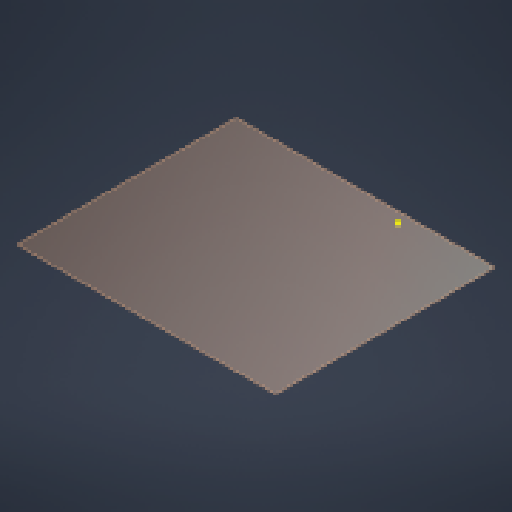
# Autodesk Inventor part: Cover Right
Saved by Autodesk Inventor 2026.1 (Build 301233020, 233B)
## iProperties
Created: 2026-06-25
Part Number: Cover Right
Material: Generic
Document SubType Name: Modeling
Designer: Bahaa
Mass: 5.68876 g
Surface Area: 120.492 cm^2
Volume: 5.68876 cm^3
Density: 1 g/cm^3
Appearance: Black PLA
Author: Bahaa
Autodesk Inventor part; units mm, degrees
ref_plane "YZ Plane" through (0, 0, 0) normal (1, 0, 0) x (0, 1, 0)
ref_plane "XZ Plane" through (0, 0, 0) normal (0, 1, 0) x (-1, 0, 0)
ref_plane "XY Plane" through (0, 0, 0) normal (0, 0, 1) x (1, 0, 0)
ref_plane "Work Plane1" through (0, 0, 0) normal (0, 0, 1) x (1, 0, 0)
sketch "Sketch1" plane through (0, 0, 0) normal (0, 0, 1) x (1, 0, 0)
  circle A0 centre (-1.9788, -172.3545) radius 2.85 projected
  circle A1 centre (36.7695, -114.5513) radius 1.6 projected
  circle A2 centre (-114.5513, -114.5513) radius 1.6 projected
  circle A3 centre (-114.5513, -36.7695) radius 1.6 projected
  circle A4 centre (36.7696, -36.7696) radius 1.6 projected
  circle A5 centre (-120.2082, -108.8944) radius 2.85 projected
  circle A6 centre (-120.2082, -42.4264) radius 2.85 projected
  circle A7 centre (42.4264, -42.4264) radius 2.85 projected
  circle A8 centre (42.4264, -108.8944) radius 2.85 projected
  circle A9 centre (0, -151.3209) radius 2.85 projected
  circle A10 centre (-77.7818, -151.3208) radius 2.85 projected
  arc A11 (3.1213, -2.5355) -> (3.3245, -2.9609) centre (3.2981, -2.7123) ccw projected
  arc A12 (4.9497, -3.5355) -> (3.3245, -2.9609) centre (3.5355, -4.9497) ccw projected
  line L0 (4.9497, -3.5355) -> (33.234, -31.8198) projected
  arc A13 (33.234, -34.6482) -> (33.234, -31.8198) centre (31.8198, -33.234) ccw projected
  line L1 (33.234, -34.6482) -> (32.5269, -35.3553) projected
  arc A14 (32.5269, -35.3553) -> (32.5269, -38.1838) centre (33.9411, -36.7696) ccw projected
  line L2 (32.5269, -38.1838) -> (41.0122, -46.669) projected
  arc A15 (41.0122, -46.669) -> (43.8406, -46.669) centre (42.4264, -45.2548) ccw projected
  line L3 (43.8406, -46.669) -> (50.8531, -39.6566) projected
  arc A16 (54.1372, -40.3613) -> (50.8531, -39.6566) centre (52.2673, -41.0708) ccw projected
  arc A17 (54.1372, -110.9596) -> (54.1372, -40.3613) centre (-38.8909, -75.6604) ccw projected
  arc A18 (50.8531, -111.6643) -> (54.1372, -110.9596) centre (52.2673, -110.25) ccw projected
  line L4 (50.8531, -111.6643) -> (43.8406, -104.6518) projected
  arc A19 (43.8406, -104.6518) -> (41.0122, -104.6518) centre (42.4264, -106.066) ccw projected
  line L5 (41.0122, -104.6518) -> (32.5269, -113.1371) projected
  arc A20 (32.5269, -113.1371) -> (32.5269, -115.9655) centre (33.9411, -114.5513) ccw projected
  line L6 (32.5269, -115.9655) -> (33.234, -116.6726) projected
  arc A21 (33.234, -119.501) -> (33.234, -116.6726) centre (31.8198, -118.0868) ccw projected
  line L7 (33.234, -119.501) -> (4.9497, -147.7853) projected
  arc A22 (2.1213, -147.7853) -> (4.9497, -147.7853) centre (3.5355, -146.3711) ccw projected
  line L8 (2.1213, -147.7853) -> (1.4142, -147.0782) projected
  arc A23 (1.4142, -147.0782) -> (-1.4142, -147.0782) centre (0, -148.4924) ccw projected
  line L9 (-1.4142, -147.0782) -> (-9.8995, -155.5635) projected
  arc A24 (-9.8995, -155.5635) -> (-9.8995, -158.3919) centre (-8.4853, -156.9777) ccw projected
  line L10 (-9.8995, -158.3919) -> (-2.8871, -165.4044) projected
  arc A25 (-3.5917, -168.6885) -> (-2.8871, -165.4044) centre (-4.3013, -166.8186) ccw projected
  arc A26 (-21.3624, -173.6043) -> (-3.5917, -168.6885) centre (-38.8909, -75.6604) ccw projected
  arc A27 (-24.8909, -170.6512) -> (-21.3624, -173.6043) centre (-21.8909, -170.6512) ccw projected
  line L11 (-24.8909, -107.6604) -> (-24.8909, -170.6512) projected
  arc A28 (-24.8909, -107.6604) -> (-27.8909, -104.6604) centre (-27.8909, -107.6604) ccw projected
  line L12 (-49.8909, -104.6604) -> (-27.8909, -104.6604) projected
  arc A29 (-49.8909, -104.6604) -> (-52.8909, -107.6604) centre (-49.8909, -107.6604) ccw projected
  line L13 (-52.8909, -170.6512) -> (-52.8909, -107.6604) projected
  arc A30 (-56.4194, -173.6043) -> (-52.8909, -170.6512) centre (-55.8909, -170.6512) ccw projected
  arc A31 (-74.19, -168.6885) -> (-56.4194, -173.6043) centre (-38.8909, -75.6604) ccw projected
  arc A32 (-74.8947, -165.4044) -> (-74.19, -168.6885) centre (-73.4805, -166.8186) ccw projected
  line L14 (-74.8947, -165.4044) -> (-67.8823, -158.3919) projected
  arc A33 (-67.8823, -158.3919) -> (-67.8823, -155.5635) centre (-69.2965, -156.9777) ccw projected
  line L15 (-67.8823, -155.5635) -> (-76.3675, -147.0782) projected
  arc A34 (-76.3675, -147.0782) -> (-79.196, -147.0782) centre (-77.7817, -148.4924) ccw projected
  line L16 (-79.196, -147.0782) -> (-79.9031, -147.7853) projected
  arc A35 (-82.7315, -147.7853) -> (-79.9031, -147.7853) centre (-81.3173, -146.3711) ccw projected
  line L17 (-82.7315, -147.7853) -> (-111.0158, -119.501) projected
  arc A36 (-111.0158, -116.6726) -> (-111.0158, -119.501) centre (-109.6016, -118.0868) ccw projected
  line L18 (-111.0158, -116.6726) -> (-110.3087, -115.9655) projected
  arc A37 (-110.3087, -115.9655) -> (-110.3087, -113.1371) centre (-111.7229, -114.5513) ccw projected
  line L19 (-110.3087, -113.1371) -> (-118.794, -104.6518) projected
  arc A38 (-118.794, -104.6518) -> (-121.6224, -104.6518) centre (-120.2082, -106.066) ccw projected
  line L20 (-121.6224, -104.6518) -> (-128.6348, -111.6642) projected
  arc A39 (-131.9189, -110.9596) -> (-128.6348, -111.6642) centre (-130.049, -110.25) ccw projected
  arc A40 (-138.0344, -84.0758) -> (-131.9189, -110.9596) centre (-38.8909, -75.6604) ccw projected
  arc A41 (-138.0344, -84.0758) -> (-139.0308, -83.1604) centre (-139.0308, -84.1604) ccw projected
  line L21 (-139.0308, -83.1604) -> (-143.8909, -83.1604) projected
  arc A42 (-144.8909, -82.1604) -> (-143.8909, -83.1604) centre (-143.8909, -82.1604) ccw projected
  line L22 (-144.8909, -82.1604) -> (-144.8909, -69.1604) projected
  arc A43 (-143.8909, -68.1604) -> (-144.8909, -69.1604) centre (-143.8909, -69.1604) ccw projected
  line L23 (-143.8909, -68.1604) -> (-139.0308, -68.1604) projected
  arc A44 (-139.0308, -68.1604) -> (-138.0344, -67.245) centre (-139.0308, -67.1604) ccw projected
  arc A45 (-131.9189, -40.3613) -> (-138.0344, -67.245) centre (-38.8909, -75.6604) ccw projected
  arc A46 (-128.6348, -39.6566) -> (-131.9189, -40.3613) centre (-130.049, -41.0708) ccw projected
  line L24 (-128.6348, -39.6566) -> (-121.6224, -46.669) projected
  arc A47 (-121.6224, -46.669) -> (-118.7939, -46.669) centre (-120.2082, -45.2548) ccw projected
  line L25 (-118.7939, -46.669) -> (-110.3087, -38.1838) projected
  arc A48 (-110.3087, -38.1838) -> (-110.3087, -35.3553) centre (-111.7229, -36.7696) ccw projected
  line L26 (-110.3087, -35.3553) -> (-111.0158, -34.6482) projected
  arc A49 (-111.0158, -31.8198) -> (-111.0158, -34.6482) centre (-109.6016, -33.234) ccw projected
  line L27 (-111.0158, -31.8198) -> (-82.7315, -3.5355) projected
  arc A50 (-81.1062, -2.9609) -> (-82.7315, -3.5355) centre (-81.3173, -4.9497) ccw projected
  arc A51 (-81.1062, -2.9609) -> (-80.9031, -2.5355) centre (-81.0798, -2.7123) ccw projected
  line L28 (-80.9031, -2.5355) -> (-83.4386, 0) projected
  line L29 (-83.4386, 0) -> (-119.8546, -36.416) projected
  arc A52 (-120.5617, -36.416) -> (-119.8546, -36.416) centre (-120.2082, -36.0624) ccw projected
  line L30 (-120.5617, -36.416) -> (-131.6714, -25.3063) projected
  arc A53 (-131.6714, -25.3063) -> (-134.06, -25.6695) centre (-132.732, -26.367) ccw projected
  arc A54 (-134.06, -25.6695) -> (-134.06, -125.6514) centre (-38.8909, -75.6604) ccw projected
  arc A55 (-134.06, -125.6514) -> (-131.6714, -126.0145) centre (-132.732, -124.9538) ccw projected
  line L31 (-131.6714, -126.0145) -> (-120.5617, -114.9048) projected
  arc A56 (-119.8546, -114.9048) -> (-120.5617, -114.9048) centre (-120.2082, -115.2584) ccw projected
  line L32 (-119.8546, -114.9048) -> (-78.1353, -156.6241) projected
  arc A57 (-78.1353, -157.3312) -> (-78.1353, -156.6241) centre (-78.4889, -156.9777) ccw projected
  line L33 (-78.1353, -157.3312) -> (-89.245, -168.4409) projected
  arc A58 (-89.245, -168.4409) -> (-88.8818, -170.8295) centre (-88.1843, -169.5016) ccw projected
  arc A59 (-88.8818, -170.8295) -> (-52.1373, -182.3412) centre (-38.8909, -75.6604) ccw projected
  arc A60 (-52.1373, -182.3412) -> (-49.8909, -180.3564) centre (-51.8909, -180.3564) ccw projected
  line L34 (-49.8909, -108.6604) -> (-49.8909, -180.3564) projected
  arc A61 (-48.8909, -107.6604) -> (-49.8909, -108.6604) centre (-48.8909, -108.6604) ccw projected
  line L35 (-28.8909, -107.6604) -> (-48.8909, -107.6604) projected
  arc A62 (-27.8909, -108.6604) -> (-28.8909, -107.6604) centre (-28.8909, -108.6604) ccw projected
  line L36 (-27.8909, -108.6604) -> (-27.8909, -180.3564) projected
  arc A63 (-27.8909, -180.3564) -> (-25.6444, -182.3412) centre (-25.8909, -180.3564) ccw projected
  arc A64 (-25.6444, -182.3412) -> (11.1001, -170.8295) centre (-38.8909, -75.6604) ccw projected
  arc A65 (11.1001, -170.8295) -> (11.4632, -168.4409) centre (10.4025, -169.5016) ccw projected
  line L37 (11.4632, -168.4409) -> (0.3535, -157.3313) projected
  arc A66 (0.3535, -156.6242) -> (0.3535, -157.3313) centre (0.7071, -156.9777) ccw projected
  line L38 (0.3535, -156.6242) -> (42.0728, -114.9049) projected
  arc A67 (42.7799, -114.9049) -> (42.0728, -114.9049) centre (42.4264, -115.2584) ccw projected
  line L39 (42.7799, -114.9049) -> (53.8896, -126.0145) projected
  arc A68 (53.8896, -126.0145) -> (56.2782, -125.6514) centre (54.9503, -124.9538) ccw projected
  arc A69 (56.2782, -125.6514) -> (56.2782, -25.6695) centre (-38.8909, -75.6604) ccw projected
  arc A70 (56.2782, -25.6695) -> (53.8896, -25.3064) centre (54.9503, -26.367) ccw projected
  line L40 (53.8896, -25.3064) -> (42.78, -36.416) projected
  arc A71 (42.0729, -36.416) -> (42.78, -36.416) centre (42.4264, -36.0624) ccw projected
  line L41 (42.0729, -36.416) -> (5.6568, 0) projected
  line L42 (5.6568, 0) -> (3.1213, -2.5355) projected
  arc A72 (-22.8909, -107.6604) -> (-27.8909, -102.6604) centre (-27.8909, -107.6604) ccw
  line L43 (-22.8909, -107.6604) -> (-22.8909, -170.6512)
  arc A73 (-22.8909, -170.6512) -> (-21.7147, -171.6356) centre (-21.8909, -170.6512) ccw
  arc A74 (-21.7147, -171.6356) -> (-4.3013, -166.8186) centre (-38.8909, -75.6604) ccw
  line L44 (-4.3013, -166.8186) -> (-11.3137, -159.8061)
  arc A75 (-11.3137, -154.1493) -> (-11.3137, -159.8061) centre (-8.4853, -156.9777) ccw
  line L45 (-11.3137, -154.1493) -> (-2.8284, -145.664)
  arc A76 (2.8284, -145.664) -> (-2.8284, -145.664) centre (0, -148.4924) ccw
  line L46 (2.8284, -145.664) -> (3.5355, -146.3711)
  line L47 (3.5355, -146.3711) -> (31.8198, -118.0868)
  line L48 (31.8198, -118.0868) -> (31.1127, -117.3797)
  arc A77 (31.1127, -111.7229) -> (31.1127, -117.3797) centre (33.9411, -114.5513) ccw
  line L49 (31.1127, -111.7229) -> (39.598, -103.2376)
  arc A78 (45.2548, -103.2376) -> (39.598, -103.2376) centre (42.4264, -106.066) ccw
  line L50 (45.2548, -103.2376) -> (52.2673, -110.25)
  arc A79 (52.2673, -110.25) -> (52.2673, -41.0708) centre (-38.8909, -75.6604) ccw
  line L51 (52.2673, -41.0708) -> (45.2548, -48.0833)
  arc A80 (39.598, -48.0833) -> (45.2548, -48.0833) centre (42.4264, -45.2548) ccw
  line L52 (39.598, -48.0833) -> (31.1127, -39.598)
  arc A81 (31.1127, -33.9411) -> (31.1127, -39.598) centre (33.9411, -36.7696) ccw
  line L53 (31.1127, -33.9411) -> (31.8198, -33.234)
  line L54 (31.8198, -33.234) -> (3.5355, -4.9497)
  arc A82 (1.7071, -1.1213) -> (3.5355, -4.9497) centre (3.2981, -2.7123) ccw
  line L55 (1.7071, -1.1213) -> (5.6568, 2.8284)
  line L56 (5.6568, 2.8284) -> (42.4264, -33.9411)
  line L57 (42.4264, -33.9411) -> (52.4754, -23.8921)
  arc A83 (58.0488, -24.7394) -> (52.4754, -23.8921) centre (54.9503, -26.367) ccw
  arc A84 (58.0488, -126.5815) -> (58.0488, -24.7394) centre (-38.8909, -75.6604) ccw
  arc A85 (52.4754, -127.4287) -> (58.0488, -126.5815) centre (54.9503, -124.9538) ccw
  line L58 (52.4754, -127.4287) -> (42.4264, -117.3797)
  line L59 (42.4264, -117.3797) -> (2.8284, -156.9777)
  line L60 (2.8284, -156.9777) -> (12.8774, -167.0267)
  arc A86 (12.0301, -172.6001) -> (12.8774, -167.0267) centre (10.4025, -169.5016) ccw
  arc A87 (-25.398, -184.3259) -> (12.0301, -172.6001) centre (-38.8909, -75.6604) ccw
  arc A88 (-29.8909, -180.3564) -> (-25.398, -184.3259) centre (-25.8909, -180.3564) ccw
  line L61 (-29.8909, -180.3564) -> (-29.8909, -109.6604)
  line L62 (-29.8909, -109.6604) -> (-47.8909, -109.6604)
  line L63 (-47.8909, -109.6604) -> (-47.8909, -180.3564)
  arc A89 (-52.3838, -184.3259) -> (-47.8909, -180.3564) centre (-51.8909, -180.3564) ccw
  arc A90 (-89.8119, -172.6001) -> (-52.3838, -184.3259) centre (-38.8909, -75.6604) ccw
  arc A91 (-90.6592, -167.0267) -> (-89.8119, -172.6001) centre (-88.1843, -169.5016) ccw
  line L64 (-90.6592, -167.0267) -> (-80.6102, -156.9777)
  line L65 (-80.6102, -156.9777) -> (-120.2082, -117.3797)
  line L66 (-120.2082, -117.3797) -> (-130.2571, -127.4287)
  arc A92 (-135.8306, -126.5814) -> (-130.2571, -127.4287) centre (-132.732, -124.9538) ccw
  arc A93 (-135.8305, -24.7394) -> (-135.8306, -126.5814) centre (-38.8909, -75.6604) ccw
  arc A94 (-130.2571, -23.8921) -> (-135.8305, -24.7394) centre (-132.732, -26.367) ccw
  line L67 (-130.2571, -23.8921) -> (-120.2082, -33.9411)
  line L68 (-120.2082, -33.9411) -> (-83.4386, 2.8284)
  line L69 (-83.4386, 2.8284) -> (-79.4889, -1.1213)
  arc A95 (-81.3173, -4.9497) -> (-79.4889, -1.1213) centre (-81.0798, -2.7123) ccw
  line L70 (-81.3173, -4.9497) -> (-109.6016, -33.234)
  line L71 (-109.6016, -33.234) -> (-108.8945, -33.9411)
  arc A96 (-108.8945, -39.598) -> (-108.8945, -33.9411) centre (-111.7229, -36.7696) ccw
  line L72 (-108.8945, -39.598) -> (-117.3797, -48.0832)
  arc A97 (-123.0366, -48.0832) -> (-117.3797, -48.0832) centre (-120.2082, -45.2548) ccw
  line L73 (-123.0366, -48.0832) -> (-130.049, -41.0708)
  arc A98 (-130.049, -41.0708) -> (-136.0415, -67.4141) centre (-38.8909, -75.6604) ccw
  arc A99 (-139.0308, -70.1604) -> (-136.0415, -67.4141) centre (-139.0308, -67.1604) ccw
  line L74 (-139.0308, -70.1604) -> (-142.8909, -70.1604)
  line L75 (-142.8909, -70.1604) -> (-142.8909, -81.1604)
  line L76 (-142.8909, -81.1604) -> (-139.0308, -81.1604)
  arc A100 (-136.0415, -83.9067) -> (-139.0308, -81.1604) centre (-139.0308, -84.1604) ccw
  arc A101 (-136.0415, -83.9067) -> (-130.049, -110.25) centre (-38.8909, -75.6604) ccw
  line L77 (-130.049, -110.25) -> (-123.0366, -103.2376)
  arc A102 (-117.3797, -103.2376) -> (-123.0366, -103.2376) centre (-120.2082, -106.066) ccw
  line L78 (-117.3797, -103.2376) -> (-108.8945, -111.7229)
  arc A103 (-108.8945, -117.3797) -> (-108.8945, -111.7229) centre (-111.7229, -114.5513) ccw
  line L79 (-108.8945, -117.3797) -> (-109.6016, -118.0868)
  line L80 (-109.6016, -118.0868) -> (-81.3173, -146.3711)
  line L81 (-81.3173, -146.3711) -> (-80.6102, -145.664)
  arc A104 (-74.9533, -145.664) -> (-80.6102, -145.664) centre (-77.7817, -148.4924) ccw
  line L82 (-74.9533, -145.664) -> (-66.4681, -154.1493)
  arc A105 (-66.4681, -159.8061) -> (-66.4681, -154.1493) centre (-69.2965, -156.9777) ccw
  line L83 (-66.4681, -159.8061) -> (-73.4805, -166.8186)
  arc A106 (-73.4805, -166.8186) -> (-56.067, -171.6356) centre (-38.8909, -75.6604) ccw
  arc A107 (-56.067, -171.6356) -> (-54.8909, -170.6512) centre (-55.8909, -170.6512) ccw
  line L84 (-54.8909, -170.6512) -> (-54.8909, -107.6604)
  arc A108 (-49.8909, -102.6604) -> (-54.8909, -107.6604) centre (-49.8909, -107.6604) ccw
  line L85 (-49.8909, -102.6604) -> (-27.8909, -102.6604)
  line L86 (26.5165, -25.1023) -> (18.0312, -33.5876)
  line L87 (30.052, -24.3952) -> (19.4454, -35.0018)
  line L88 (19.4454, -35.0018) -> (-48.2132, -102.6604)
  line L89 (-22.8909, -107.6604) -> (-22.8909, -93.6016)
  line L90 (-22.8909, -93.6016) -> (-22.8909, -183.9852)
  circle A109 centre (-38.8909, -63.6604) radius 1.35 projected
  circle A110 centre (-38.8909, -87.6604) radius 1.35 projected
  arc A111 (-134.1409, -64.6604) -> (-136.1409, -66.6604) centre (-134.1409, -66.6604) ccw projected
  line L91 (-136.1409, -84.6604) -> (-136.1409, -66.6604) projected
  arc A112 (-136.1409, -84.6604) -> (-134.1409, -86.6604) centre (-134.1409, -84.6604) ccw projected
  line L92 (-113.1409, -86.6604) -> (-134.1409, -86.6604) projected
  arc A113 (-111.1409, -88.6604) -> (-113.1409, -86.6604) centre (-113.1409, -88.6604) ccw projected
  line L93 (-111.1409, -89.9104) -> (-111.1409, -88.6604) projected
  arc A114 (-111.1409, -89.9104) -> (-109.1409, -91.9104) centre (-109.1409, -89.9104) ccw projected
  line L94 (-3.8909, -91.9104) -> (-109.1409, -91.9104) projected
  arc A115 (-1.8948, -93.7854) -> (-3.8909, -91.9104) centre (-3.8909, -93.9104) ccw projected
  arc A116 (-1.8948, -93.7854) -> (0.1013, -95.6604) centre (0.1013, -93.6604) ccw projected
  line L95 (45.1169, -95.6604) -> (0.1013, -95.6604) projected
  arc A117 (45.1169, -95.6604) -> (47.113, -93.7854) centre (45.1169, -93.6604) ccw projected
  arc A118 (49.1091, -91.9104) -> (47.113, -93.7854) centre (49.1091, -93.9104) ccw projected
  line L96 (55.1091, -91.9104) -> (49.1091, -91.9104) projected
  arc A119 (55.1091, -91.9104) -> (57.1091, -89.9104) centre (55.1091, -89.9104) ccw projected
  line L97 (57.1091, -57.6604) -> (57.1091, -89.9104) projected
  arc A120 (57.1091, -57.6604) -> (55.1091, -55.6604) centre (55.1091, -57.6604) ccw projected
  line L98 (0.1091, -55.6604) -> (55.1091, -55.6604) projected
  arc A121 (0.1091, -55.6604) -> (-1.887, -57.5354) centre (0.1091, -57.6604) ccw projected
  arc A122 (-3.8831, -59.4104) -> (-1.887, -57.5354) centre (-3.8831, -57.4104) ccw projected
  line L99 (-106.6409, -59.4104) -> (-3.8831, -59.4104) projected
  arc A123 (-106.6409, -59.4104) -> (-108.6409, -61.4104) centre (-106.6409, -61.4104) ccw projected
  line L100 (-108.6409, -62.6604) -> (-108.6409, -61.4104) projected
  arc A124 (-110.6409, -64.6604) -> (-108.6409, -62.6604) centre (-110.6409, -62.6604) ccw projected
  line L101 (-134.1409, -64.6604) -> (-110.6409, -64.6604) projected
  arc A125 (59.1091, -57.6604) -> (55.1091, -53.6604) centre (55.1091, -57.6604) ccw
  line L102 (59.1091, -57.6604) -> (59.1091, -89.9104)
  arc A126 (55.1091, -93.9104) -> (59.1091, -89.9104) centre (55.1091, -89.9104) ccw
  line L103 (55.1091, -93.9104) -> (49.1091, -93.9104)
  arc A127 (45.1169, -97.6604) -> (49.1091, -93.9104) centre (45.1169, -93.6604) ccw
  line L104 (45.1169, -97.6604) -> (0.1013, -97.6604)
  arc A128 (-3.8909, -93.9104) -> (0.1013, -97.6604) centre (0.1013, -93.6604) ccw
  line L105 (-3.8909, -93.9104) -> (-109.1409, -93.9104)
  arc A129 (-113.1409, -89.9104) -> (-109.1409, -93.9104) centre (-109.1409, -89.9104) ccw
  line L106 (-113.1409, -89.9104) -> (-113.1409, -88.6604)
  line L107 (-113.1409, -88.6604) -> (-134.1409, -88.6604)
  arc A130 (-138.1409, -84.6604) -> (-134.1409, -88.6604) centre (-134.1409, -84.6604) ccw
  line L108 (-138.1409, -84.6604) -> (-138.1409, -66.6604)
  arc A131 (-134.1409, -62.6604) -> (-138.1409, -66.6604) centre (-134.1409, -66.6604) ccw
  line L109 (-134.1409, -62.6604) -> (-110.6409, -62.6604)
  line L110 (-110.6409, -62.6604) -> (-110.6409, -61.4104)
  arc A132 (-106.6409, -57.4104) -> (-110.6409, -61.4104) centre (-106.6409, -61.4104) ccw
  line L111 (-106.6409, -57.4104) -> (-3.8831, -57.4104)
  arc A133 (0.1091, -53.6604) -> (-3.8831, -57.4104) centre (0.1091, -57.6604) ccw
  line L112 (0.1091, -53.6604) -> (55.1091, -53.6604)
  point P0 (0, 0)
  point P1 (-22.8909, -93.9104)
  point P2 (-22.8909, -181.9631)
  point P3 (0.7868, -53.6604)
  dimension "d0" = 2
  dimension "d1" = 2
  dimension "d2" = 2
  constraints: 118 end point, 93 point on circle, 46 centre point, 3 point on line, 1 parallel, 1 vertical, 101 other
  measures "d0" radial gap between concentric circles of A28 A72
  measures "d1" distance between parallel lines of L86 L87
  measures "d2" distance between parallel lines of L98 L112
extrude "Extrusion1" add sketch "Sketch1" along normal blind 1 contours L41 A71 L40 A70 A69 A68 L39 A67 L38 A66 L37 A65 A64 L90 A27 A26 A25 L10 A24 L9 A23 L8 A22 L7 A21 L6 A20 L5 A19 L4 A18 A17 L102 A125 A16 L3 A15 L2 A14 L1 A13 L0 L87 | L0 A13 L1 A14 L2 A15 L3 A16 A17 A125 A79 L51 A80 L52 A81 L53 L54 L87 | L54 L53 A81 L52 A80 L51 A79 A125 L112 L88 L87 | L105 A128 L104 A127 L103 A126 A79 L50 A78 L49 A77 L48 L47 L46 A76 L45 A75 L44 A74 A73 L43 L89 | A17 A18 L4 A19 L5 A20 L6 A21 L7 A22 L8 A23 L9 A24 L10 A25 A26 A27 L90 A73 A74 L44 A75 L45 A76 L46 L47 L48 A77 L49 A78 L50 A79 A126 L102
fillet "Fillet1" radius 1 6 edges at (-22.8909, -93.9104, 0.5) (-3.8909, -93.9104, 0.5) (49.1091, -93.9104, 0.5) (0.7868, -53.6604, 0.5) (30.052, -24.3952, 0.5) (-22.8909, -181.9631, 0.5)
body "Solid1"
